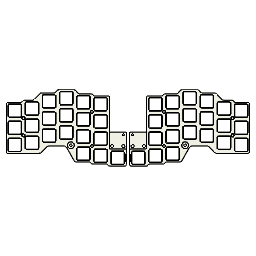
mriya-top-plate-fdm-v1.03 (Autodesk Fusion 360 design; units mm, degrees)
Autodesk Fusion 360 part; units mm, degrees
sketch "mriya-top-plate" plane through (0, 0, 0) normal (0, 0, 1) x (1, 0, 0)
  arc A0 (-117.8, 77.3932) -> (-119.9, 79.4932) centre (-119.9, 77.3932) ccw
  line L0 (-132.4, 59.0932) -> (-132.4, 46.6932)
  line L1 (-114, 60.4932) -> (-114, 49.6932)
  arc A1 (-131.6, 78.8932) -> (-132.4, 78.0932) centre (-131.6, 78.0932) ccw
  line L2 (-131.6, 59.8932) -> (-119.2, 59.8932)
  circle A2 centre (-115.9, 63.5432) radius 1.45
  line L3 (-117.8, 58.3932) -> (-117.8, 47.5932)
  line L4 (-130.9, 60.4932) -> (-119.9, 60.4932)
  arc A3 (-131.6, 59.8932) -> (-132.4, 59.0932) centre (-131.6, 59.0932) ccw
  line L5 (-130.9, 79.4932) -> (-119.9, 79.4932)
  arc A4 (-119.2, 64.8932) -> (-118.4, 65.6932) centre (-119.2, 65.6932) ccw
  line L6 (-130.9, 64.2932) -> (-120.1, 64.2932)
  line L7 (-134.6, 79.4932) -> (-134.6, 26.2932) construction
  line L8 (-133, 77.3932) -> (-133, 66.3932)
  line L9 (-117.8, 77.3932) -> (-117.8, 66.5932)
  line L10 (-131.6, 78.8932) -> (-119.2, 78.8932)
  line L11 (-106.1426, 83.2932) -> (-115.0716, 83.2932) construction
  arc A5 (-115.0716, 83.2932) -> (-116.4858, 82.7074) centre (-115.0716, 81.2933) ccw construction
  arc A6 (-119.0284, 80.9932) -> (-117.6142, 81.579) centre (-119.0284, 82.9932) ccw construction
  arc A7 (-118.4, 59.0932) -> (-119.2, 59.8932) centre (-119.2, 59.0932) ccw
  arc A8 (-133, 66.3932) -> (-130.9, 64.2932) centre (-130.9, 66.3932) ccw
  line L12 (-133, 58.3932) -> (-133, 47.3932)
  line L13 (-113.4, 61.3932) -> (-113.4, 48.9932)
  arc A9 (-133.1, 80.9932) -> (-134.6, 79.4932) centre (-133.1, 79.4932) ccw construction
  line L14 (-74.6, 40.6932) -> (-62.2, 40.6932)
  line L15 (-73.9, 40.0932) -> (-62.9, 40.0932)
  line L16 (-73.9, 78.0932) -> (-62.9, 78.0932)
  arc A10 (-134.6, 26.2932) -> (-133.1, 24.7932) centre (-133.1, 26.2932) ccw construction
  arc A11 (-131.6, 40.8932) -> (-132.4, 40.0932) centre (-131.6, 40.0932) ccw
  arc A12 (-130.9, 41.4932) -> (-133, 39.3932) centre (-130.9, 39.3932) ccw
  arc A13 (-119.2, 26.8932) -> (-118.4, 27.6932) centre (-119.2, 27.6932) ccw
  line L17 (-73.9, 55.2932) -> (-62.9, 55.2932)
  line L18 (-74.6, 54.6932) -> (-62.2, 54.6932)
  arc A14 (-114, 30.6932) -> (-111.9, 28.5932) centre (-111.9, 30.6932) ccw
  line L19 (-113.4, 42.3932) -> (-113.4, 29.9932)
  line L20 (-130.9, 26.2932) -> (-119.9, 26.2932)
  arc A15 (-119.9, 26.2932) -> (-117.8, 28.3932) centre (-119.9, 28.3932) ccw
  line L21 (-74.6, 92.6932) -> (-62.2, 92.6932)
  line L22 (-132.4, 40.0932) -> (-132.4, 27.6932)
  arc A16 (-113.4, 29.9932) -> (-112.6, 29.1932) centre (-112.6, 29.9932) ccw
  line L23 (-130.9, 41.4932) -> (-119.9, 41.4932)
  arc A17 (-118.4, 40.0932) -> (-119.2, 40.8932) centre (-119.2, 40.0932) ccw
  line L24 (-77.0716, 94.7932) -> (-59.7284, 94.7932) construction
  line L25 (-114, 41.4932) -> (-114, 30.6932)
  arc A18 (-132.4, 27.6932) -> (-131.6, 26.8932) centre (-131.6, 27.6932) ccw
  arc A19 (-133, 28.3932) -> (-130.9, 26.2932) centre (-130.9, 28.3932) ccw
  line L26 (-117.8, 39.3932) -> (-117.8, 28.3932)
  line L27 (-131.6, 40.8932) -> (-119.2, 40.8932)
  line L28 (-73.9, 59.0932) -> (-62.9, 59.0932)
  arc A20 (-117.8, 39.3932) -> (-119.9, 41.4932) centre (-119.9, 39.3932) ccw
  line L29 (-131.6, 26.8932) -> (-119.2, 26.8932)
  line L30 (-74.6, 78.6932) -> (-62.2, 78.6932)
  line L31 (-112.6, 29.1932) -> (-100.2, 29.1932)
  line L32 (-111.9, 66.5932) -> (-100.9, 66.5932)
  line L33 (-130.9, 45.2932) -> (-120.1, 45.2932)
  arc A21 (-133, 47.3932) -> (-130.9, 45.2932) centre (-130.9, 47.3932) ccw
  line L34 (-112.6, 62.1932) -> (-100.2, 62.1932)
  arc A22 (-120.1, 45.2932) -> (-117.8, 47.5932) centre (-120.1, 47.5932) ccw
  arc A23 (-119.2, 45.8932) -> (-118.4, 46.6932) centre (-119.2, 46.6932) ccw
  line L35 (-133.1, 24.7932) -> (-98.1426, 24.7932) construction
  line L36 (-131.6, 45.8932) -> (-119.2, 45.8932)
  arc A24 (-132.4, 46.6932) -> (-131.6, 45.8932) centre (-131.6, 46.6932) ccw
  line L37 (-111.7, 62.7932) -> (-100.9, 62.7932)
  circle A25 centre (-63.3, 33.4932) radius 1.4
  arc A26 (-114, 49.6932) -> (-111.9, 47.5932) centre (-111.9, 49.6932) ccw
  line L38 (-111.9, 47.5932) -> (-100.9, 47.5932)
  arc A27 (-111.7, 43.7932) -> (-114, 41.4932) centre (-111.7, 41.4932) ccw
  circle A28 centre (-63.3, 33.4932) radius 3.8
  line L39 (-133, 39.3932) -> (-133, 28.3932)
  line L40 (-74.6, 73.6932) -> (-62.2, 73.6932)
  line L41 (-118.4, 40.0932) -> (-118.4, 27.6932)
  arc A29 (-113.4, 48.9932) -> (-112.6, 48.1932) centre (-112.6, 48.9932) ccw
  circle A30 centre (-115.9, 44.5432) radius 1.45
  line L42 (-74.6, 59.6932) -> (-62.2, 59.6932)
  line L43 (-112.6, 81.1932) -> (-100.2, 81.1932)
  line L44 (-118.4, 59.0932) -> (-118.4, 46.6932)
  line L45 (-111.7, 43.7932) -> (-100.9, 43.7932)
  arc A31 (-113.4, 67.9932) -> (-112.6, 67.1932) centre (-112.6, 67.9932) ccw
  arc A32 (-111.9, 81.7932) -> (-114, 79.6932) centre (-111.9, 79.6932) ccw
  line L46 (-111.9, 81.7932) -> (-100.9, 81.7932)
  arc A33 (-114, 68.6932) -> (-111.9, 66.5932) centre (-111.9, 68.6932) ccw
  line L47 (-112.6, 43.1932) -> (-100.2, 43.1932)
  arc A34 (-111.7, 62.7932) -> (-114, 60.4932) centre (-111.7, 60.4932) ccw
  arc A35 (-112.6, 81.1932) -> (-113.4, 80.3932) centre (-112.6, 80.3932) ccw
  arc A36 (-106.1426, 83.2932) -> (-104.0213, 84.1719) centre (-106.1426, 86.2932) ccw construction
  line L48 (-114, 79.6932) -> (-114, 68.6932)
  line L49 (-112.6, 48.1932) -> (-100.2, 48.1932)
  line L50 (-112.6, 67.1932) -> (-100.2, 67.1932)
  line L51 (-111.9, 28.5932) -> (-100.9, 28.5932)
  line L52 (-113.4, 80.3932) -> (-113.4, 67.9932)
  arc A37 (-112.6, 62.1932) -> (-113.4, 61.3932) centre (-112.6, 61.3932) ccw
  line L53 (-104.0213, 84.1719) -> (-97.4858, 90.7074) construction
  arc A38 (-10.1, 30.7932) -> (-10.1, 34.1932) centre (-10.1, 32.4932) ccw construction
  line L54 (-36.6, 33.8932) -> (-24.2, 33.8932)
  arc A39 (-43.2, 17.1932) -> (-42.4, 17.9932) centre (-43.2, 17.9932) ccw
  line L55 (-36.6, 28.8932) -> (-24.2, 28.8932)
  line L56 (-35.9, 14.2932) -> (-24.9, 14.2932)
  arc A40 (-62.9, 40.0932) -> (-60.8, 42.1932) centre (-62.9, 42.1932) ccw
  line L57 (-55.6, 31.1932) -> (-43.2, 31.1932)
  arc A41 (-43.9, 35.5932) -> (-41.8, 37.6932) centre (-43.9, 37.6932) ccw
  line L58 (-35.7, 33.2932) -> (-24.9, 33.2932)
  arc A42 (-56.4, 17.9932) -> (-55.6, 17.1932) centre (-55.6, 17.9932) ccw
  line L59 (-54.9, 16.5932) -> (-43.9, 16.5932)
  arc A43 (-43.2, 36.1932) -> (-42.4, 36.9932) centre (-43.2, 36.9932) ccw
  arc A44 (-41.8, 29.4932) -> (-44.1, 31.7932) centre (-44.1, 29.4932) ccw
  arc A45 (-41.6142, 14.5074) -> (-43.0284, 15.0932) centre (-43.0284, 13.0933) ccw construction
  arc A46 (-43.9, 16.5932) -> (-41.8, 18.6932) centre (-43.9, 18.6932) ccw
  arc A47 (-42.4, 30.3932) -> (-43.2, 31.1932) centre (-43.2, 30.3932) ccw
  line L60 (-35.9, 29.4932) -> (-24.9, 29.4932)
  line L61 (-36.6, 14.8932) -> (-24.2, 14.8932)
  line L62 (-21.4858, 11.079) -> (-22.6142, 12.2074) construction
  arc A48 (-4.4, 25.7932) -> (-5.2, 26.5932) centre (-5.2, 25.7932) ccw
  line L63 (-18.4, 25.7932) -> (-18.4, 13.3932)
  line L64 (-17.6, 26.5932) -> (-5.2, 26.5932)
  line L65 (-16.9, 27.1932) -> (-5.7, 27.1932)
  line L66 (-4, 25.4932) -> (-4, 13.6932)
  line L67 (-4.4, 25.7932) -> (-4.4, 13.3932)
  line L68 (-2.75, 23.6932) -> (-2.75, 15.4932)
  arc A49 (-24.9, 14.2932) -> (-22.8, 16.3932) centre (-24.9, 16.3932) ccw
  line L69 (-17.6, 12.5932) -> (-5.2, 12.5932)
  circle A50 centre (-17.6, 32.4932) radius 1.7
  line L70 (-19, 25.0932) -> (-19, 14.0932)
  line L71 (-2.1, 11.9932) -> (-2.1, 28.6932) construction
  arc A51 (-17.6, 26.5932) -> (-18.4, 25.7932) centre (-17.6, 25.7932) ccw
  circle A52 centre (-5.1, 45.1932) radius 1.1
  arc A53 (-5.2, 12.5932) -> (-4.4, 13.3932) centre (-5.2, 13.3932) ccw
  arc A54 (-5.7, 11.9932) -> (-4, 13.6932) centre (-5.7, 13.6932) ccw
  arc A55 (-3.6, 10.4932) -> (-2.1, 11.9932) centre (-3.6, 11.9932) ccw construction
  arc A56 (-12.7, 34.1932) -> (-12.7, 30.7932) centre (-12.7, 32.4932) ccw construction
  line L72 (-22.8, 27.3932) -> (-22.8, 16.3932)
  arc A57 (-19, 14.0932) -> (-16.9, 11.9932) centre (-16.9, 14.0932) ccw
  arc A58 (-36.6, 28.8932) -> (-37.4, 28.0932) centre (-36.6, 28.0932) ccw
  arc A59 (-37.4, 15.6932) -> (-36.6, 14.8932) centre (-36.6, 15.6932) ccw
  circle A60 centre (-39.9, 32.5432) radius 1.45
  arc A61 (-21.4858, 11.079) -> (-20.0716, 10.4932) centre (-20.0716, 12.4932) ccw construction
  line L73 (-23.4, 28.0932) -> (-23.4, 15.6932)
  arc A62 (-24.2, 14.8932) -> (-23.4, 15.6932) centre (-24.2, 15.6932) ccw
  arc A63 (-16.9, 27.1932) -> (-19, 25.0932) centre (-16.9, 25.0932) ccw
  line L74 (-16.9, 11.9932) -> (-5.7, 11.9932)
  arc A64 (-23.4, 28.0932) -> (-24.2, 28.8932) centre (-24.2, 28.0932) ccw
  arc A65 (-22.8, 27.3932) -> (-24.9, 29.4932) centre (-24.9, 27.3932) ccw
  arc A66 (-2.1, 28.6932) -> (-2.9, 29.4932) centre (-2.9, 28.6932) ccw construction
  arc A67 (-18.4, 13.3932) -> (-17.6, 12.5932) centre (-17.6, 13.3932) ccw
  arc A68 (-4, 25.4932) -> (-5.7, 27.1932) centre (-5.7, 25.4932) ccw
  line L75 (-3.6, 10.4932) -> (-20.0716, 10.4932) construction
  arc A69 (-22.6142, 12.2074) -> (-24.0284, 12.7932) centre (-24.0284, 10.7933) ccw construction
  arc A70 (-22.8, 84.3932) -> (-24.9, 86.4932) centre (-24.9, 84.3932) ccw
  arc A71 (-37.4, 53.6932) -> (-36.6, 52.8932) centre (-36.6, 53.6932) ccw
  line L76 (-20.7, 49.1932) -> (-20.7, 87.3632)
  arc A72 (-35.9, 67.4932) -> (-38, 65.3932) centre (-35.9, 65.3932) ccw
  arc A73 (-35.9, 48.4932) -> (-38, 46.3932) centre (-35.9, 46.3932) ccw
  line L77 (-54.9, 50.7932) -> (-43.9, 50.7932)
  line L78 (-22.8, 84.3932) -> (-22.8, 73.3932)
  arc A74 (-60.8, 53.1932) -> (-62.9, 55.2932) centre (-62.9, 53.1932) ccw
  arc A75 (-24.9, 52.2932) -> (-22.8, 54.3932) centre (-24.9, 54.3932) ccw
  arc A76 (-42.4, 49.3932) -> (-43.2, 50.1932) centre (-43.2, 49.3932) ccw
  arc A77 (-41.8, 48.6932) -> (-43.9, 50.7932) centre (-43.9, 48.6932) ccw
  line L79 (-1.93, 29.4932) -> (-20.7, 29.4932)
  line L80 (-12.7, 34.1932) -> (-10.1, 34.1932) construction
  arc A78 (-24.9, 33.2932) -> (-22.8, 35.3932) centre (-24.9, 35.3932) ccw
  line L81 (-10.1, 30.7932) -> (-12.7, 30.7932) construction
  circle A79 centre (-11.4, 32.4932) radius 1.15 construction
  line L82 (-19.7, 29.4932) -> (-2.9, 29.4932) construction
  circle A80 centre (-5.1, 32.4932) radius 1.7
  arc A81 (-24.2, 33.8932) -> (-23.4, 34.6932) centre (-24.2, 34.6932) ccw
  arc A82 (-37.4, 34.6932) -> (-36.6, 33.8932) centre (-36.6, 34.6932) ccw
  arc A83 (-40.4858, 13.379) -> (-39.0716, 12.7932) centre (-39.0716, 14.7932) ccw construction
  arc A84 (-35.9, 29.4932) -> (-38, 27.3932) centre (-35.9, 27.3932) ccw
  arc A85 (-38, 35.5932) -> (-35.7, 33.2932) centre (-35.7, 35.5932) ccw
  arc A86 (-38, 16.3932) -> (-35.9, 14.2932) centre (-35.9, 16.3932) ccw
  line L83 (-37.4, 28.0932) -> (-37.4, 15.6932)
  arc A87 (-58.3142, 94.2074) -> (-59.7284, 94.7932) centre (-59.7284, 92.7932) ccw construction
  line L84 (-61.4, 72.8932) -> (-61.4, 60.4932)
  line L85 (-36.6, 66.8932) -> (-24.2, 66.8932)
  line L86 (-35.7, 71.2932) -> (-24.9, 71.2932)
  line L87 (-54.9, 73.5932) -> (-43.9, 73.5932)
  line L88 (-54.9, 88.7932) -> (-43.9, 88.7932)
  line L89 (-35.9, 52.2932) -> (-24.9, 52.2932)
  arc A88 (-54.9, 88.7932) -> (-57, 86.6932) centre (-54.9, 86.6932) ccw
  line L90 (-61.4, 91.8932) -> (-61.4, 79.4932)
  line L91 (-56.4, 87.3932) -> (-56.4, 74.9932)
  arc A89 (-61.4, 91.8932) -> (-62.2, 92.6932) centre (-62.2, 91.8932) ccw
  line L92 (-55.6, 88.1932) -> (-43.2, 88.1932)
  line L93 (-55.6, 74.1932) -> (-43.2, 74.1932)
  line L94 (-60.8, 72.1932) -> (-60.8, 61.1932)
  arc A90 (-57, 75.6932) -> (-54.9, 73.5932) centre (-54.9, 75.6932) ccw
  circle A91 centre (-39.9, 70.5432) radius 1.45
  arc A92 (-54.9858, 90.879) -> (-53.5716, 90.2932) centre (-53.5716, 92.2931) ccw construction
  arc A93 (-38, 73.5932) -> (-35.7, 71.2932) centre (-35.7, 73.5932) ccw
  arc A94 (-62.9, 78.0932) -> (-60.8, 80.1932) centre (-62.9, 80.1932) ccw
  arc A95 (-56.4, 74.9932) -> (-55.6, 74.1932) centre (-55.6, 74.9932) ccw
  line L95 (-53.5716, 90.2932) -> (-40.7284, 90.2932) construction
  arc A96 (-62.2, 78.6932) -> (-61.4, 79.4932) centre (-62.2, 79.4932) ccw
  line L96 (-57, 86.6932) -> (-57, 75.6932)
  arc A97 (-60.8, 91.1932) -> (-62.9, 93.2932) centre (-62.9, 91.1932) ccw
  arc A98 (-39.3142, 89.7074) -> (-40.7284, 90.2932) centre (-40.7284, 88.2932) ccw construction
  line L97 (-37.4, 85.0932) -> (-37.4, 72.6932)
  arc A99 (-55.6, 88.1932) -> (-56.4, 87.3932) centre (-55.6, 87.3932) ccw
  arc A100 (-60.8, 72.1932) -> (-62.9, 74.2932) centre (-62.9, 72.1932) ccw
  arc A101 (-61.4, 72.8932) -> (-62.2, 73.6932) centre (-62.2, 72.8932) ccw
  line L98 (-60.8, 91.1932) -> (-60.8, 80.1932)
  line L99 (-58.3142, 94.2074) -> (-54.9858, 90.879) construction
  line L100 (-38.1858, 88.579) -> (-39.3142, 89.7074) construction
  line L101 (-99.4, 42.3932) -> (-99.4, 29.9932)
  arc A102 (-81.2, 37.1932) -> (-80.4, 37.9932) centre (-81.2, 37.9932) ccw
  arc A103 (-75.4, 41.4932) -> (-74.6, 40.6932) centre (-74.6, 41.4932) ccw
  line L102 (-96.0213, 25.6719) -> (-89.7787, 31.9145) construction
  arc A104 (-76, 42.1932) -> (-73.9, 40.0932) centre (-73.9, 42.1932) ccw
  line L103 (-42.4, 49.3932) -> (-42.4, 36.9932)
  arc A105 (-94.4, 37.9932) -> (-93.6, 37.1932) centre (-93.6, 37.9932) ccw
  arc A106 (-67.7517, 30.7608) -> (-71.2344, 32.7932) centre (-71.2344, 28.793) ccw construction
  line L104 (-98.8, 41.6932) -> (-98.8, 30.6932)
  arc A107 (-98.1426, 24.7932) -> (-96.0213, 25.6719) centre (-98.1426, 27.7931) ccw construction
  arc A108 (-87.6574, 32.7932) -> (-89.7787, 31.9145) centre (-87.6573, 29.7931) ccw construction
  arc A109 (-99.4, 42.3932) -> (-100.2, 43.1932) centre (-100.2, 42.3932) ccw
  line L105 (-20.7, 29.4932) -> (-20.7, 49.1932)
  line L106 (-36.6, 52.8932) -> (-24.2, 52.8932)
  line L107 (-57, 48.6932) -> (-57, 37.6932)
  circle A110 centre (-5.1, 45.1932) radius 2.2 construction
  line L108 (-35.9, 86.4932) -> (-24.9, 86.4932)
  line L109 (-60.8, 53.1932) -> (-60.8, 42.1932)
  line L110 (-36.7716, 87.9932) -> (-21.5, 87.9932) construction
  line L111 (-23.4, 47.0932) -> (-23.4, 34.6932)
  line L112 (-36.6, 47.8932) -> (-24.2, 47.8932)
  line L113 (-35.9, 48.4932) -> (-24.9, 48.4932)
  line L114 (-36.6, 85.8932) -> (-24.2, 85.8932)
  line L115 (-41.8, 48.6932) -> (-41.8, 37.6932)
  line L116 (-37.4, 47.0932) -> (-37.4, 34.6932)
  line L117 (-36.6, 71.8932) -> (-24.2, 71.8932)
  line L118 (-56.4, 49.3932) -> (-56.4, 36.9932)
  line L119 (-22.8, 46.3932) -> (-22.8, 35.3932)
  line L120 (-38, 46.3932) -> (-38, 35.5932)
  line L121 (-20.7, 30.4932) -> (-20.7, 87.1932) construction
  line L122 (-35.9, 67.4932) -> (-24.9, 67.4932)
  line L123 (-61.4, 53.8932) -> (-61.4, 41.4932)
  line L124 (-95, 68.6932) -> (-95, 57.6932)
  line L125 (-75.4, 72.8932) -> (-75.4, 60.4932)
  line L126 (-79.8, 68.6932) -> (-79.8, 57.6932)
  line L127 (-80.4, 69.3932) -> (-80.4, 56.9932)
  arc A111 (-82.2284, 91.2932) -> (-80.8142, 91.879) centre (-82.2284, 93.2932) ccw construction
  arc A112 (-79.8, 68.6932) -> (-81.9, 70.7932) centre (-81.9, 68.6932) ccw
  line L128 (-76, 72.1932) -> (-76, 61.1932)
  line L129 (-94.4, 69.3932) -> (-94.4, 56.9932)
  arc A113 (-112.6, 43.1932) -> (-113.4, 42.3932) centre (-112.6, 42.3932) ccw
  line L130 (-76, 91.1932) -> (-76, 80.1932)
  arc A114 (-73.9, 93.2932) -> (-76, 91.1932) centre (-73.9, 91.1932) ccw
  arc A115 (-76, 80.1932) -> (-73.9, 78.0932) centre (-73.9, 80.1932) ccw
  arc A116 (-92.9, 89.7932) -> (-95, 87.6932) centre (-92.9, 87.6932) ccw
  line L131 (-78.4858, 94.2074) -> (-80.8142, 91.879) construction
  arc A117 (-73.9, 74.2932) -> (-76, 72.1932) centre (-73.9, 72.1932) ccw
  arc A118 (-74.6, 73.6932) -> (-75.4, 72.8932) centre (-74.6, 72.8932) ccw
  line L132 (-79.8, 87.6932) -> (-79.8, 76.6932)
  arc A119 (-75.4, 79.4932) -> (-74.6, 78.6932) centre (-74.6, 79.4932) ccw
  line L133 (-59.4741, 16.1094) -> (-67.7517, 30.7608) construction
  line L134 (-80.4, 88.3932) -> (-80.4, 75.9932)
  line L135 (-75.4, 91.8932) -> (-75.4, 79.4932)
  arc A120 (-77.0716, 94.7932) -> (-78.4858, 94.2074) centre (-77.0716, 92.7933) ccw construction
  arc A121 (-94.4, 75.9932) -> (-93.6, 75.1932) centre (-93.6, 75.9932) ccw
  arc A122 (-100.2, 67.1932) -> (-99.4, 67.9932) centre (-100.2, 67.9932) ccw
  line L136 (-93.6, 89.1932) -> (-81.2, 89.1932)
  arc A123 (-100.9, 66.5932) -> (-98.8, 68.6932) centre (-100.9, 68.6932) ccw
  arc A124 (-96.0716, 91.2932) -> (-97.4858, 90.7074) centre (-96.0716, 89.2933) ccw construction
  line L137 (-99.4, 80.3932) -> (-99.4, 67.9932)
  arc A125 (-92.9, 70.7932) -> (-95, 68.6932) centre (-92.9, 68.6932) ccw
  line L138 (-92.9, 89.7932) -> (-81.9, 89.7932)
  line L139 (-93.6, 70.1932) -> (-81.2, 70.1932)
  line L140 (-95, 87.6932) -> (-95, 76.6932)
  arc A126 (-99.4, 80.3932) -> (-100.2, 81.1932) centre (-100.2, 80.3932) ccw
  line L141 (-92.9, 70.7932) -> (-81.9, 70.7932)
  line L142 (-92.9, 74.5932) -> (-81.9, 74.5932)
  line L143 (-94.4, 88.3932) -> (-94.4, 75.9932)
  line L144 (-93.6, 75.1932) -> (-81.2, 75.1932)
  arc A127 (-93.6, 89.1932) -> (-94.4, 88.3932) centre (-93.6, 88.3932) ccw
  arc A128 (-98.8, 79.6932) -> (-100.9, 81.7932) centre (-100.9, 79.6932) ccw
  arc A129 (-93.6, 70.1932) -> (-94.4, 69.3932) centre (-93.6, 69.3932) ccw
  arc A130 (-80.4, 88.3932) -> (-81.2, 89.1932) centre (-81.2, 88.3932) ccw
  line L145 (-96.0716, 91.2932) -> (-82.2284, 91.2932) construction
  arc A131 (-95, 76.6932) -> (-92.9, 74.5932) centre (-92.9, 76.6932) ccw
  arc A132 (-79.8, 87.6932) -> (-81.9, 89.7932) centre (-81.9, 87.6932) ccw
  line L146 (-98.8, 79.6932) -> (-98.8, 68.6932)
  arc A133 (-81.9, 74.5932) -> (-79.8, 76.6932) centre (-81.9, 76.6932) ccw
  arc A134 (-80.4, 69.3932) -> (-81.2, 70.1932) centre (-81.2, 69.3932) ccw
  arc A135 (-81.2, 75.1932) -> (-80.4, 75.9932) centre (-81.2, 75.9932) ccw
  arc A136 (-20.7, 30.4932) -> (-19.7, 29.4932) centre (-19.7, 30.4932) ccw construction
  line L147 (-54.9, 35.5932) -> (-43.9, 35.5932)
  line L148 (-43.0284, 15.0932) -> (-57.7328, 15.0932) construction
  line L149 (-55.6, 17.1932) -> (-43.2, 17.1932)
  line L150 (-55.6, 36.1932) -> (-43.2, 36.1932)
  arc A137 (-57, 18.6932) -> (-54.9, 16.5932) centre (-54.9, 18.6932) ccw
  line L151 (-73.9, 74.2932) -> (-62.9, 74.2932)
  line L152 (-57, 29.6932) -> (-57, 18.6932)
  line L153 (-73.9, 93.2932) -> (-62.9, 93.2932)
  line L154 (-38, 27.3932) -> (-38, 16.3932)
  line L155 (-41.8, 29.4932) -> (-41.8, 18.6932)
  line L156 (-56.4, 30.3932) -> (-56.4, 17.9932)
  arc A138 (-55.6, 31.1932) -> (-56.4, 30.3932) centre (-55.6, 30.3932) ccw
  arc A139 (-57, 37.6932) -> (-54.9, 35.5932) centre (-54.9, 37.6932) ccw
  arc A140 (-54.9, 31.7932) -> (-57, 29.6932) centre (-54.9, 29.6932) ccw
  arc A141 (-59.4741, 16.1094) -> (-57.7328, 15.0932) centre (-57.7328, 17.0932) ccw construction
  line L157 (-40.4858, 13.379) -> (-41.6142, 14.5074) construction
  arc A142 (-56.4, 36.9932) -> (-55.6, 36.1932) centre (-55.6, 36.9932) ccw
  line L158 (-54.9, 31.7932) -> (-44.1, 31.7932)
  line L159 (-42.4, 30.3932) -> (-42.4, 17.9932)
  arc A143 (-62.2, 40.6932) -> (-61.4, 41.4932) centre (-62.2, 41.4932) ccw
  arc A144 (-93.6, 51.1932) -> (-94.4, 50.3932) centre (-93.6, 50.3932) ccw
  line L160 (-93.6, 37.1932) -> (-81.2, 37.1932)
  arc A145 (-81.9, 36.5932) -> (-79.8, 38.6932) centre (-81.9, 38.6932) ccw
  arc A146 (-95, 57.6932) -> (-92.9, 55.5932) centre (-92.9, 57.6932) ccw
  arc A147 (-79.8, 49.6932) -> (-81.9, 51.7932) centre (-81.9, 49.6932) ccw
  arc A148 (-94.4, 56.9932) -> (-93.6, 56.1932) centre (-93.6, 56.9932) ccw
  arc A149 (-100.2, 29.1932) -> (-99.4, 29.9932) centre (-100.2, 29.9932) ccw
  arc A150 (-98.8, 41.6932) -> (-100.9, 43.7932) centre (-100.9, 41.6932) ccw
  arc A151 (-95, 38.6932) -> (-92.9, 36.5932) centre (-92.9, 38.6932) ccw
  arc A152 (-100.2, 48.1932) -> (-99.4, 48.9932) centre (-100.2, 48.9932) ccw
  arc A153 (-100.9, 47.5932) -> (-98.8, 49.6932) centre (-100.9, 49.6932) ccw
  line L161 (-92.9, 55.5932) -> (-81.9, 55.5932)
  arc A154 (-100.9, 28.5932) -> (-98.8, 30.6932) centre (-100.9, 30.6932) ccw
  line L162 (-87.6574, 32.7932) -> (-71.2344, 32.7932) construction
  line L163 (-92.9, 36.5932) -> (-81.9, 36.5932)
  arc A155 (-76, 61.1932) -> (-73.9, 59.0932) centre (-73.9, 61.1932) ccw
  line L164 (-93.6, 51.1932) -> (-81.2, 51.1932)
  arc A156 (-92.9, 51.7932) -> (-95, 49.6932) centre (-92.9, 49.6932) ccw
  line L165 (-94.4, 50.3932) -> (-94.4, 37.9932)
  arc A157 (-75.4, 60.4932) -> (-74.6, 59.6932) centre (-74.6, 60.4932) ccw
  arc A158 (-73.9, 55.2932) -> (-76, 53.1932) centre (-73.9, 53.1932) ccw
  line L166 (-98.8, 60.6932) -> (-98.8, 49.6932)
  arc A159 (-80.4, 50.3932) -> (-81.2, 51.1932) centre (-81.2, 50.3932) ccw
  line L167 (-93.6, 56.1932) -> (-81.2, 56.1932)
  arc A160 (-81.2, 56.1932) -> (-80.4, 56.9932) centre (-81.2, 56.9932) ccw
  line L168 (-79.8, 49.6932) -> (-79.8, 38.6932)
  arc A161 (-81.9, 55.5932) -> (-79.8, 57.6932) centre (-81.9, 57.6932) ccw
  line L169 (-75.4, 53.8932) -> (-75.4, 41.4932)
  line L170 (-99.4, 61.3932) -> (-99.4, 48.9932)
  arc A162 (-98.8, 60.6932) -> (-100.9, 62.7932) centre (-100.9, 60.6932) ccw
  arc A163 (-74.6, 92.6932) -> (-75.4, 91.8932) centre (-74.6, 91.8932) ccw
  line L171 (-80.4, 50.3932) -> (-80.4, 37.9932)
  arc A164 (-74.6, 54.6932) -> (-75.4, 53.8932) centre (-74.6, 53.8932) ccw
  arc A165 (-99.4, 61.3932) -> (-100.2, 62.1932) centre (-100.2, 61.3932) ccw
  line L172 (-95, 49.6932) -> (-95, 38.6932)
  line L173 (-76, 53.1932) -> (-76, 42.1932)
  line L174 (-92.9, 51.7932) -> (-81.9, 51.7932)
  line L175 (-23.4, 66.0932) -> (-23.4, 53.6932)
  arc A166 (-23.4, 85.0932) -> (-24.2, 85.8932) centre (-24.2, 85.0932) ccw
  arc A167 (-20.7, 49.1932) -> (-19.7, 48.1932) centre (-19.7, 49.1932) ccw
  arc A168 (-22.8, 65.3932) -> (-24.9, 67.4932) centre (-24.9, 65.3932) ccw
  arc A169 (-24.9, 71.2932) -> (-22.8, 73.3932) centre (-24.9, 73.3932) ccw
  line L176 (-39.0716, 12.7932) -> (-24.0284, 12.7932) construction
  arc A170 (-24.2, 71.8932) -> (-23.4, 72.6932) centre (-24.2, 72.6932) ccw
  arc A171 (-23.4, 47.0932) -> (-24.2, 47.8932) centre (-24.2, 47.0932) ccw
  line L177 (-23.4, 85.0932) -> (-23.4, 72.6932)
  arc A172 (-22.8, 46.3932) -> (-24.9, 48.4932) centre (-24.9, 46.3932) ccw
  line L178 (-22.8, 65.3932) -> (-22.8, 54.3932)
  line L179 (-19.7, 48.1932) -> (-2.73, 48.1932)
  arc A173 (-20.7, 87.1932) -> (-21.5, 87.9932) centre (-21.5, 87.1932) ccw construction
  arc A174 (-24.2, 52.8932) -> (-23.4, 53.6932) centre (-24.2, 53.6932) ccw
  arc A175 (-23.4, 66.0932) -> (-24.2, 66.8932) centre (-24.2, 66.0932) ccw
  line L180 (-42.4, 68.3932) -> (-42.4, 55.9932)
  arc A176 (-36.6, 85.8932) -> (-37.4, 85.0932) centre (-36.6, 85.0932) ccw
  arc A177 (-43.2, 74.1932) -> (-42.4, 74.9932) centre (-43.2, 74.9932) ccw
  arc A178 (-38.1858, 88.579) -> (-36.7716, 87.9932) centre (-36.7716, 89.9932) ccw construction
  arc A179 (-61.4, 53.8932) -> (-62.2, 54.6932) centre (-62.2, 53.8932) ccw
  arc A180 (-37.4, 72.6932) -> (-36.6, 71.8932) centre (-36.6, 72.6932) ccw
  arc A181 (-36.6, 47.8932) -> (-37.4, 47.0932) centre (-36.6, 47.0932) ccw
  arc A182 (-43.9, 73.5932) -> (-41.8, 75.6932) centre (-43.9, 75.6932) ccw
  arc A183 (-35.9, 86.4932) -> (-38, 84.3932) centre (-35.9, 84.3932) ccw
  line L181 (-41.8, 86.6932) -> (-41.8, 75.6932)
  line L182 (-37.4, 66.0932) -> (-37.4, 53.6932)
  arc A184 (-54.9, 50.7932) -> (-57, 48.6932) centre (-54.9, 48.6932) ccw
  arc A185 (-41.8, 86.6932) -> (-43.9, 88.7932) centre (-43.9, 86.6932) ccw
  line L183 (-57, 67.6932) -> (-57, 56.6932)
  line L184 (-38, 84.3932) -> (-38, 73.5932)
  arc A186 (-57, 56.6932) -> (-54.9, 54.5932) centre (-54.9, 56.6932) ccw
  arc A187 (-42.4, 87.3932) -> (-43.2, 88.1932) centre (-43.2, 87.3932) ccw
  line L185 (-42.4, 87.3932) -> (-42.4, 74.9932)
  arc A188 (-55.6, 69.1932) -> (-56.4, 68.3932) centre (-55.6, 68.3932) ccw
  arc A189 (-54.9, 69.7932) -> (-57, 67.6932) centre (-54.9, 67.6932) ccw
  line L186 (-54.9, 69.7932) -> (-44.1, 69.7932)
  line L187 (-55.6, 55.1932) -> (-43.2, 55.1932)
  line L188 (-55.6, 50.1932) -> (-43.2, 50.1932)
  arc A190 (-62.2, 59.6932) -> (-61.4, 60.4932) centre (-62.2, 60.4932) ccw
  line L189 (-41.8, 67.4932) -> (-41.8, 56.6932)
  arc A191 (-56.4, 55.9932) -> (-55.6, 55.1932) centre (-55.6, 55.9932) ccw
  arc A192 (-41.8, 67.4932) -> (-44.1, 69.7932) centre (-44.1, 67.4932) ccw
  arc A193 (-43.9, 54.5932) -> (-41.8, 56.6932) centre (-43.9, 56.6932) ccw
  arc A194 (-43.2, 55.1932) -> (-42.4, 55.9932) centre (-43.2, 55.9932) ccw
  line L190 (-56.4, 68.3932) -> (-56.4, 55.9932)
  arc A195 (-55.6, 50.1932) -> (-56.4, 49.3932) centre (-55.6, 49.3932) ccw
  arc A196 (-62.9, 59.0932) -> (-60.8, 61.1932) centre (-62.9, 61.1932) ccw
  arc A197 (-36.6, 66.8932) -> (-37.4, 66.0932) centre (-36.6, 66.0932) ccw
  line L191 (-55.6, 69.1932) -> (-43.2, 69.1932)
  arc A198 (-42.4, 68.3932) -> (-43.2, 69.1932) centre (-43.2, 68.3932) ccw
  arc A199 (-38, 54.3932) -> (-35.9, 52.2932) centre (-35.9, 54.3932) ccw
  line L192 (-54.9, 54.5932) -> (-43.9, 54.5932)
  line L193 (-38, 65.3932) -> (-38, 54.3932)
  arc A200 (-130.9, 60.4932) -> (-133, 58.3932) centre (-130.9, 58.3932) ccw
  arc A201 (-120.1, 64.2932) -> (-117.8, 66.5932) centre (-120.1, 66.5932) ccw
  line L194 (-131.6, 64.8932) -> (-119.2, 64.8932)
  line L195 (-132.4, 78.0932) -> (-132.4, 65.6932)
  line L196 (-118.4, 78.0932) -> (-118.4, 65.6932)
  line L197 (-117.6142, 81.579) -> (-116.4858, 82.7074) construction
  arc A202 (-117.8, 58.3932) -> (-119.9, 60.4932) centre (-119.9, 58.3932) ccw
  line L198 (-133.1, 80.9932) -> (-119.0284, 80.9932) construction
  arc A203 (-118.4, 78.0932) -> (-119.2, 78.8932) centre (-119.2, 78.0932) ccw
  arc A204 (-130.9, 79.4932) -> (-133, 77.3932) centre (-130.9, 77.3932) ccw
  arc A205 (-132.4, 65.6932) -> (-131.6, 64.8932) centre (-131.6, 65.6932) ccw
  arc A206 (-58.194, 94.3276) -> (-59.7284, 94.9632) centre (-59.7284, 92.7932) ccw
  line L199 (-77.0716, 94.9632) -> (-59.7284, 94.9632)
  arc A207 (-77.0716, 94.9632) -> (-78.606, 94.3276) centre (-77.0716, 92.7933) ccw
  line L200 (-78.606, 94.3276) -> (-80.9344, 91.9992)
  arc A208 (-82.2284, 91.4632) -> (-80.9344, 91.9992) centre (-82.2284, 93.2932) ccw
  line L201 (-96.0716, 91.4632) -> (-82.2284, 91.4632)
  arc A209 (-96.0716, 91.4632) -> (-97.606, 90.8276) centre (-96.0716, 89.2933) ccw
  line L202 (-104.1415, 84.2921) -> (-97.606, 90.8276)
  arc A210 (-106.1426, 83.4632) -> (-104.1415, 84.2921) centre (-106.1426, 86.2932) ccw
  line L203 (-106.1426, 83.4632) -> (-115.0716, 83.4632)
  arc A211 (-115.0716, 83.4632) -> (-116.606, 82.8276) centre (-115.0716, 81.2933) ccw
  line L204 (-117.7344, 81.6992) -> (-116.606, 82.8276)
  arc A212 (-119.0284, 81.1632) -> (-117.7344, 81.6992) centre (-119.0284, 82.9932) ccw
  line L205 (-133.1, 81.1632) -> (-119.0284, 81.1632)
  arc A213 (-133.1, 81.1632) -> (-134.77, 79.4932) centre (-133.1, 79.4932) ccw
  line L206 (-134.77, 79.4932) -> (-134.77, 26.2932)
  arc A214 (-134.77, 26.2932) -> (-133.1, 24.6232) centre (-133.1, 26.2932) ccw
  line L207 (-133.1, 24.6232) -> (-98.1426, 24.6232)
  arc A215 (-98.1426, 24.6232) -> (-95.9011, 25.5517) centre (-98.1426, 27.7931) ccw
  line L208 (-95.9011, 25.5517) -> (-89.6585, 31.7943)
  arc A216 (-87.6574, 32.6232) -> (-89.6585, 31.7943) centre (-87.6573, 29.7931) ccw
  line L209 (-87.6574, 32.6232) -> (-71.2344, 32.6232)
  arc A217 (-67.8997, 30.6772) -> (-71.2344, 32.6232) centre (-71.2344, 28.793) ccw
  line L210 (-59.6221, 16.0258) -> (-67.8997, 30.6772)
  arc A218 (-59.6221, 16.0258) -> (-57.7328, 14.9232) centre (-57.7328, 17.0932) ccw
  line L211 (-43.0284, 14.9232) -> (-57.7328, 14.9232)
  arc A219 (-41.7344, 14.3872) -> (-43.0284, 14.9232) centre (-43.0284, 13.0933) ccw
  line L212 (-40.606, 13.2588) -> (-41.7344, 14.3872)
  arc A220 (-40.606, 13.2588) -> (-39.0716, 12.6232) centre (-39.0716, 14.7932) ccw
  line L213 (-39.0716, 12.6232) -> (-24.0284, 12.6232)
  arc A221 (-22.7344, 12.0872) -> (-24.0284, 12.6232) centre (-24.0284, 10.7933) ccw
  line L214 (-21.606, 10.9588) -> (-22.7344, 12.0872)
  arc A222 (-21.606, 10.9588) -> (-20.0716, 10.3232) centre (-20.0716, 12.4932) ccw
  line L215 (-3.6, 10.3232) -> (-20.0716, 10.3232)
  arc A223 (-3.6, 10.3232) -> (-1.93, 11.9932) centre (-3.6, 11.9932) ccw
  line L216 (-1.93, 11.9932) -> (-1.93, 47.3932)
  line L217 (-36.7716, 88.1632) -> (-21.5, 88.1632)
  arc A224 (-38.0656, 88.6992) -> (-36.7716, 88.1632) centre (-36.7716, 89.9932) ccw
  line L218 (-38.0656, 88.6992) -> (-39.194, 89.8276)
  arc A225 (-39.194, 89.8276) -> (-40.7284, 90.4632) centre (-40.7284, 88.2932) ccw
  line L219 (-53.5716, 90.4632) -> (-40.7284, 90.4632)
  arc A226 (-54.8656, 90.9992) -> (-53.5716, 90.4632) centre (-53.5716, 92.2931) ccw
  line L220 (-58.194, 94.3276) -> (-54.8656, 90.9992)
  arc A227 (-20.7, 87.3632) -> (-21.5, 88.1632) centre (-21.5, 87.3632) ccw
  arc A228 (-1.93, 47.3932) -> (-2.73, 48.1932) centre (-2.73, 47.3932) ccw
  line L221 (-1.93, 15.4932) -> (-2.75, 15.4932)
  line L222 (-1.93, 23.6932) -> (-2.75, 23.6932)
  dimension "d1" = 2.9
  dimension "d2" = 2.9
  dimension "d3" = 2.8
  dimension "d4" = 2.9
  dimension "d5" = 2.9
  dimension "d6" = 3.4
  dimension "d7" = 3.4
  dimension "d8" = 7.6
  dimension "d9" = 2.3
  dimension "d10" = 2.2
  dimension "d11" = 4.4
  constraint tangent L100 A178
  constraint tangent A98 L100
  constraint tangent A92 L95
  constraint tangent A87 L99
  constraint tangent L24 A120
  constraint tangent A111 L131
  constraint tangent A124 L145
  constraint tangent A6 L197
  constraint tangent A9 L198
  constraint tangent L7 A10
  constraint tangent L35 A107
  constraint tangent L102 A108
  constraint tangent A106 L162
  constraint tangent L133 A141
  constraint tangent A45 L148
  constraint tangent A83 L157
  constraint tangent A69 L176
  constraint tangent L62 A61
  constraint tangent A55 L75
  constraint tangent L71 A55
  constraint perpendicular L71 L110
  constraint perpendicular L110 L121
  constraint perpendicular L71 L82
  constraint tangent A1 L195
  constraint tangent L10 A203
  constraint tangent A4 L196
  constraint tangent L194 A205
  constraint tangent L2 A3
  constraint tangent L2 A7
  constraint tangent A23 L44
  constraint tangent L36 A24
  constraint tangent A11 L27
  constraint tangent A17 L27
  constraint tangent A13 L41
  constraint tangent A18 L29
  constraint tangent L19 A16
  constraint tangent L31 A149
  constraint tangent L101 A109
  constraint tangent L47 A113
  constraint tangent L49 A152
  constraint tangent A29 L49
  constraint tangent L13 A37
  constraint tangent L34 A165
  constraint tangent A31 L50
  constraint tangent L50 A122
  constraint tangent A122 L137
  constraint tangent L137 A126
  constraint tangent L43 A35
  constraint tangent L143 A127
  constraint tangent L136 A130
  constraint tangent L134 A135
  constraint tangent A121 L144
  constraint tangent L139 A129
  constraint tangent L139 A134
  constraint tangent L127 A160
  constraint tangent A148 L167
  constraint tangent A144 L164
  constraint tangent A105 L165
  constraint tangent A105 L160
  constraint tangent A102 L160
  constraint tangent A159 L171
  constraint tangent A103 L169
  constraint tangent L14 A103
  constraint tangent L169 A164
  constraint tangent L18 A179
  constraint tangent L123 A143
  constraint tangent L42 A190
  constraint tangent L42 A157
  constraint tangent L125 A118
  constraint tangent L40 A101
  constraint tangent L30 A96
  constraint tangent L30 A119
  constraint tangent L135 A163
  constraint tangent L21 A89
  constraint tangent L91 A99
  constraint tangent L91 A95
  constraint tangent L93 A95
  constraint tangent L93 A177
  constraint tangent A177 L185
  constraint tangent A187 L185
  constraint tangent L92 A187
  constraint tangent L191 A198
  constraint tangent A188 L191
  constraint tangent A191 L190
  constraint tangent L187 A194
  constraint tangent A76 L188
  constraint tangent L188 A195
  constraint tangent L118 A195
  constraint tangent L118 A142
  constraint tangent L150 A142
  constraint tangent A43 L150
  constraint tangent A43 L103
  constraint tangent L57 A47
  constraint tangent L57 A138
  constraint tangent L156 A138
  constraint tangent A42 L156
  constraint tangent A39 L149
  constraint tangent A59 L83
  constraint tangent L61 A62
  constraint tangent L73 A64
  constraint tangent L55 A64
  constraint tangent L55 A58
  constraint tangent A58 L83
  constraint tangent L63 A67
  constraint tangent L69 A67
  constraint tangent L69 A53
  constraint tangent L67 A53
  constraint tangent A48 L67
  constraint tangent A48 L64
  constraint tangent L64 A51
  constraint tangent L63 A51
  constraint tangent L54 A81
  constraint tangent A81 L111
  constraint tangent L54 A82
  constraint tangent L116 A181
  constraint tangent L112 A171
  constraint tangent L106 A174
  constraint tangent L175 A174
  constraint tangent A71 L106
  constraint tangent L182 A197
  constraint tangent L85 A175
  constraint tangent L117 A170
  constraint tangent A170 L177
  constraint tangent L117 A180
  constraint tangent L97 A176
  constraint tangent L114 A166
  constraint tangent L121 A173
  constraint tangent L110 A173
  constraint tangent L53 A124
  constraint tangent L11 A5
  constraint tangent A36 L53
  constraint tangent L11 A36
  constraint horizontal L82
  constraint tangent L121 A136
  constraint tangent L82 A136
  constraint tangent A66 L82
  constraint tangent L71 A66
  constraint tangent A167 L179
  constraint tangent L76 A167
  constraint concentric A25 A28
  constraint tangent L105 A167
  constraint tangent L5 A204
  constraint tangent L8 A204
  constraint tangent A0 L5
  constraint tangent A0 L9
  constraint tangent L8 A8
  constraint tangent L6 A8
  constraint tangent L32 A123
  constraint tangent A123 L146
  constraint tangent A32 L46
  constraint tangent A32 L48
  constraint tangent L46 A128
  constraint tangent A128 L146
  constraint tangent A33 L48
  constraint tangent L32 A33
  constraint tangent L142 A133
  constraint tangent L132 A133
  constraint tangent A116 L138
  constraint tangent A116 L140
  constraint tangent L138 A132
  constraint tangent L132 A132
  constraint tangent L140 A131
  constraint tangent L142 A131
  constraint tangent L16 A94
  constraint tangent A94 L98
  constraint tangent A114 L153
  constraint tangent L130 A114
  constraint tangent A97 L153
  constraint tangent A97 L98
  constraint tangent L130 A115
  constraint tangent L16 A115
  constraint tangent L87 A182
  constraint tangent A182 L181
  constraint tangent L88 A88
  constraint tangent A88 L96
  constraint tangent L88 A185
  constraint tangent L181 A185
  constraint tangent A90 L96
  constraint tangent L87 A90
  constraint tangent L86 A169
  constraint tangent L78 A169
  constraint tangent L108 A183
  constraint tangent A183 L184
  constraint tangent A70 L108
  constraint tangent A70 L78
  constraint tangent L4 A200
  constraint tangent L12 A200
  constraint tangent L4 A202
  constraint tangent L3 A202
  constraint tangent L12 A21
  constraint tangent L33 A21
  constraint tangent L38 A153
  constraint tangent A153 L166
  constraint tangent L37 A162
  constraint tangent L166 A162
  constraint tangent L1 A26
  constraint tangent A26 L38
  constraint tangent L161 A161
  constraint tangent L126 A161
  constraint tangent A125 L141
  constraint tangent L124 A125
  constraint tangent A112 L141
  constraint tangent L126 A112
  constraint tangent L124 A146
  constraint tangent A146 L161
  constraint tangent L28 A196
  constraint tangent L94 A196
  constraint tangent A117 L151
  constraint tangent L128 A117
  constraint tangent A100 L151
  constraint tangent L94 A100
  constraint tangent L128 A155
  constraint tangent L28 A155
  constraint tangent A193 L192
  constraint tangent L189 A193
  constraint tangent A189 L186
  constraint tangent L183 A189
  constraint tangent L183 A186
  constraint tangent A186 L192
  constraint tangent A75 L89
  constraint tangent A75 L178
  constraint tangent A72 L122
  constraint tangent A72 L193
  constraint tangent L122 A168
  constraint tangent A168 L178
  constraint tangent A199 L193
  constraint tangent L89 A199
  constraint tangent L20 A15
  constraint tangent A15 L26
  constraint tangent A12 L23
  constraint tangent A12 L39
  constraint tangent L23 A20
  constraint tangent L26 A20
  constraint tangent A19 L39
  constraint tangent L20 A19
  constraint tangent L51 A154
  constraint tangent L104 A154
  constraint tangent L45 A150
  constraint tangent L104 A150
  constraint tangent A14 L25
  constraint tangent A14 L51
  constraint tangent A145 L163
  constraint tangent A145 L168
  constraint tangent A156 L174
  constraint tangent A156 L172
  constraint tangent A147 L174
  constraint tangent A147 L168
  constraint tangent A151 L172
  constraint tangent A151 L163
  constraint tangent L15 A40
  constraint tangent A40 L109
  constraint tangent L17 A158
  constraint tangent A158 L173
  constraint tangent L17 A74
  constraint tangent A74 L109
  constraint tangent A104 L173
  constraint tangent L15 A104
  constraint tangent A41 L147
  constraint tangent A41 L115
  constraint tangent L77 A184
  constraint tangent L107 A184
  constraint tangent L77 A77
  constraint tangent A77 L115
  constraint tangent L107 A139
  constraint tangent L147 A139
  constraint tangent L58 A78
  constraint tangent A78 L119
  constraint tangent A73 L113
  constraint tangent A73 L120
  constraint tangent L113 A172
  constraint tangent L119 A172
  constraint tangent L59 A46
  constraint tangent A46 L155
  constraint tangent A140 L158
  constraint tangent L152 A140
  constraint tangent A137 L152
  constraint tangent L59 A137
  constraint tangent L56 A49
  constraint tangent A49 L72
  constraint tangent L60 A84
  constraint tangent A84 L154
  constraint tangent L60 A65
  constraint tangent L72 A65
  constraint tangent A86 L154
  constraint tangent L56 A86
  constraint tangent L65 A63
  constraint tangent L70 A63
  constraint tangent L70 A57
  constraint tangent A57 L74
  constraint tangent L65 A68
  constraint tangent L66 A68
  constraint tangent L66 A54
  constraint tangent A54 L74
  constraint tangent A38 L80
  constraint tangent A56 L81
  constraint tangent L37 A34
  constraint tangent L1 A34
  constraint tangent L6 A201
  constraint tangent L9 A201
  constraint tangent L3 A22
  constraint tangent L33 A22
  constraint tangent A27 L45
  constraint tangent L25 A27
  constraint tangent L186 A192
  constraint tangent L189 A192
  constraint tangent A93 L184
  constraint tangent L86 A93
  constraint tangent A44 L158
  constraint tangent A44 L155
  constraint tangent A85 L120
  constraint tangent L58 A85
  constraint concentric A52 A110
  constraint concentric A87 A206
  constraint concentric A120 A207
  constraint concentric A111 A208
  constraint concentric A124 A209
  constraint concentric A36 A210
  constraint concentric A5 A211
  constraint concentric A6 A212
  constraint concentric A9 A213
  constraint concentric A10 A214
  constraint concentric A107 A215
  constraint concentric A108 A216
  constraint concentric A106 A217
  constraint concentric A141 A218
  constraint concentric A45 A219
  constraint concentric A83 A220
  constraint concentric A69 A221
  constraint concentric A61 A222
  constraint concentric A55 A223
  constraint concentric A178 A224
  constraint concentric A98 A225
  constraint concentric A92 A226
  constraint tangent A223 L216
  constraint tangent L211 A219
  constraint tangent A210 L203
  constraint tangent L203 A211
  constraint tangent A213 L206
  constraint tangent L206 A214
  constraint tangent A214 L207
  constraint tangent L207 A215
  constraint tangent A224 L218
  constraint tangent L218 A225
  constraint coincident L216 L79.start
  constraint tangent L217 A227
  constraint tangent L76 A227
  constraint tangent L179 A228
  constraint tangent L216 A228
  constraint coincident L216 L221.start
  constraint coincident L216 L222.start
  constraint perpendicular L71 L221
  constraint perpendicular L71 L222
  measures "d1" diameter of A2
  measures "d2" diameter of A30
  measures "d3" diameter of A25
  measures "d4" diameter of A60
  measures "d5" diameter of A91
  measures "d6" diameter of A80
  measures "d7" diameter of A50
  measures "d8" diameter of A28
  measures "d9" diameter of A79
  measures "d10" diameter of A52
  measures "d11" diameter of A110
extrude "Extrude3" add sketch "mriya-top-plate" along normal blind 5 contours L68 L76 L79 L105 A206 L199 A207 L200 A208 L201 A209 L202 A210 L203 A211 L204 A212 L205 A213 L206 A214 L207 A215 L208 A216 L209 A217 L210 A218 L211 A219 L212 A220 L213 A221 L214 A222 L215 A223 L216 L217 A224 L218 A225 L219 A226 L220 A227 L221 L222 makes body 1
extrude "Extrude4" add sketch "mriya-top-plate" along normal blind 1.5 contours A0 L5 L6 L8 L9 A8 A201 A204 | L1 L37 A26 L38 A34 A153 L166 A162 | A2 | L3 L4 L12 L33 A21 A22 A200 A202 | L15 L17 A40 A74 A104 L109 A158 L173 | L16 A94 A97 L98 L130 A114 A115 L153 | A12 L20 A15 L23 A19 L26 A20 L39 | A14 L25 A27 L45 L51 L104 A150 A154 | L28 L94 A100 L128 A117 L151 A155 A196 | L32 A32 L46 A33 L48 A123 A128 L146 | A28 | A30 | L56 L60 A49 L72 A65 A84 A86 L154 | A41 L77 A77 L107 L115 L147 A139 A184 | L58 A73 A78 A85 L113 L119 L120 A172 | L59 A44 A46 A137 L152 L155 A140 L158 | L65 L66 L70 A54 A57 A63 L74 A68 | L68 L216 L221 L222 | L79 L105 A167 L179 L216 A228 | A60 | A70 L78 L86 A93 L108 A169 A183 L184 | A72 A75 L89 L122 A168 L178 A199 L193 | L87 L88 A88 A90 L96 A182 L181 A185 | A91 | L124 L126 A112 A125 L141 A146 L161 A161 | A116 L132 L138 L140 L142 A131 A132 A133 | A145 A147 A151 L163 A156 L168 L172 L174 | L183 A186 A189 L186 L189 A192 A193 L192 bodies 1
chamfer "Chamfer2" distance 0.4 angle 45 4 edges at (-117.2519, 45.0675, 5) (-117.2519, 64.0675, 5) (-41.2519, 71.0675, 5) (-41.2519, 33.0675, 5) on bodies 1
fillet "Fillet5" radius 0.6 4 edges at (-1.93, 15.4932, 3.25) (-2.75, 15.4932, 3.25) (-2.75, 23.6932, 3.25) (-1.93, 23.6932, 3.25) on bodies 1
fillet "Fillet6" radius 1.67 1 edges at (-1.93, 29.4932, 3.25) on bodies 1
fillet "Fillet7" radius 1 1 edges at (-20.7, 29.4932, 3.25) on bodies 1
mirror "Mirror2" about plane through (0, 0, 0) normal (1, 0, 0) of bodies 1 makes body 2
named bodies: "Right", "Left"
